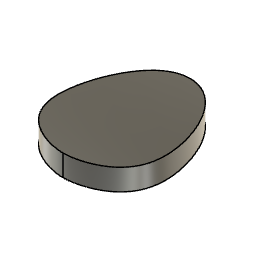
Cam v2 (Autodesk Fusion 360 design; units mm, degrees)
Autodesk Fusion 360 part; units mm, degrees
sketch "Sketch1" plane through (0, 0, 0) normal (0, 0, 1) x (1, 0, 0)
  spline S0 degree 5 poles (0, 0) (-1.0576, 0) (-3.173, 0.1256) (-6.5916, 0.6949) (-12.618, 2.46) (-20.2044, 7.356) (-25.2691, 15.5098) (-25.4975, 26.6545) (-22.7234, 38.0588) (-18.3345, 47.8428) (-12.934, 55.0734) (-6.8786, 59.3642) (-0.3337, 60.7021) (6.2933, 59.2399) (12.5651, 54.9561) (18.225, 47.7992) (22.815, 38.0711) (25.6615, 26.6223) (25.3703, 15.3737) (20.2396, 7.2241) (12.619, 2.3962) (6.59, 0.6872) (3.1727, 0.1256) (1.0576, 0) (0, 0) knots 0 0 0 0 0 0 0.05 0.1 0.15 0.2 0.25 0.3 0.35 0.4 0.45 0.5 0.55 0.6 0.65 0.7 0.75 0.8 0.85 0.9 0.95 1 1 1 1 1 1
  line L0 (-6.9446, 60.0012) -> (6.0554, 60.0012)
  line L1 (25.0707, 35.5) -> (25.0707, 10.5)
  line L2 (-24.9418, 10.5) -> (-24.9418, 35.5)
  line L3 (0, 0) -> (0, -16.5395) construction
  line L4 (0, 0) -> (56.0409, 0) construction
  line L5 (6.5, 0) -> (-6.5, 0)
  point P0 (-24.9418, 23)
  point P1 (-0.4446, 60.0012)
  point P2 (25.0707, 23)
  dimension "d1" = 13
  dimension "d2" = 25
  dimension "d3" = 25
  dimension "d4" = 13
  dimension "d5" = 23
  dimension "d6" = 23
  constraint coincident S0.start S0.end
  constraint midpoint P1 L0
  constraint midpoint P2 L1
  constraint midpoint P0 L2
  constraint vertical L3
  constraint parallel L2 L3
  constraint parallel L1 L3
  constraint perpendicular L3 L4
  constraint midpoint S0.start L5
  constraint parallel L4 L5
  constraint parallel L0 L4
  measures "d1" horizontal distance of L0.start L0.end
  measures "d2" vertical distance of L1.start L1.end
  measures "d3" vertical distance of L2.start L2.end
  measures "d4" distance of L5.start L5.end
  measures "d5" distance of P2 L4
  measures "d6" distance of P0 L4
extrude "Extrude1" add sketch "Sketch1" along normal blind 10
